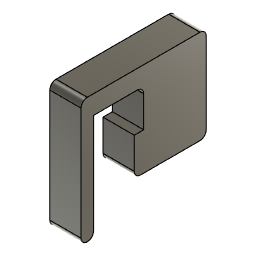
_HookF.751b9c44-9634-4196-bb50-001999120314 (Autodesk Fusion 360 design; units mm, degrees)
Autodesk Fusion 360 part; units mm, degrees
sketch "Sketch3" plane through (0, 0, 0) normal (1, 0, 0) x (0, 1, 0)
  line L0 (0, 0) -> (20, 0)
  line L1 (20, 0) -> (20, 20)
  line L2 (20, 20) -> (0, 20)
  line L3 (0, 20) -> (0, 0)
  dimension "d24" = 20
  dimension "d27" = 20
  constraint horizontal L0
  constraint vertical L1
  constraint horizontal L2
  constraint vertical L3
  constraint coincident L0.start L3.end
  measures "d24" distance of L0.start L0.end
  measures "d27" distance of L0.start L2.end
extrude "Extrude3" add sketch "Sketch3" along normal blind 5
sketch "Sketch4" plane through (5, 0, 0) normal (1, 0, 0) x (0, 1, 0)
  line L0 (0, 20) -> (0, 0)
  line L1 (0, 0) -> (20, 0)
  line L2 (20, 0) -> (20, 20)
  line L3 (20, 20) -> (0, 20)
  line L4 (2, 0) -> (2, 17)
  line L5 (2, 17) -> (10, 17)
  line L6 (10, 17) -> (10, 11)
  line L7 (10, 11) -> (8.5, 11)
  line L8 (8.5, 11) -> (8.5, 5)
  line L9 (8.5, 5) -> (20, 5)
  line L10 (20, 0) -> (2, 0)
  line L11 (20, 0) -> (20, 5)
  dimension "d30" = 8
  dimension "d31" = 2
  dimension "d32" = 6.5
  dimension "d33" = 12
  dimension "d35" = 6
  dimension "d36" = 5
  constraint coincident L1 L4.start
  constraint perpendicular L1 L4
  constraint perpendicular L2 L5
  constraint perpendicular L5 L6
  constraint perpendicular L6 L7
  constraint perpendicular L7 L8
  constraint coincident L2 L9.end
  constraint perpendicular L2 L9
  constraint coincident L1.end L2.start
  measures "d30" distance of L4.end L5.end
  measures "d31" distance of L0 L4
  measures "d32" distance of L4 L8
  measures "d33" distance of L5 L9
  measures "d35" distance of L7.end L8.end
  measures "d36" distance of L9 L10
extrude "Extrude4" cut sketch "Sketch4" against normal through all contours L1 L2 L4 L5 L6 L7 L8 L9 L10 L11
fillet "Fillet1" radius 1 7 edges at (2.5, 8.5, 5) (2.5, 10, 17) (2.5, 20, 5) (2.5, 20, 20) (2.5, 0, 20) (2.5, 0, 0) (2.5, 2, 0)
